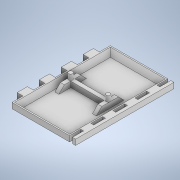
# Autodesk Inventor part: rfid_top
Saved by Autodesk Inventor 2020.1 (Build 241239000, 239)
## iProperties
Created: 2019-06-30
Part Number: rfid_top
Material: Generic
Document SubType Name: Modeling
Designer: jjsch
Density: 1 g/cm^3
Appearance: Default
Mass: 12.4406 g
Surface Area: 151.295 cm^2
Volume: 12.4406 cm^3
Author: jjsch
Autodesk Inventor part; units mm, degrees
ref_plane "YZ Plane" through (0, 0, 0) normal (1, 0, 0) x (0, 1, 0)
ref_plane "XZ Plane" through (0, 0, 0) normal (0, 1, 0) x (-1, 0, 0)
ref_plane "XY Plane" through (0, 0, 0) normal (0, 0, 1) x (1, 0, 0)
sketch "Sketch1" plane through (0, 0, 0) normal (0, 1, 0) x (-1, 0, 0)
  line L0 (-31.9185, 45) -> (31.9185, 45)
  line L1 (31.9185, 45) -> (31.9185, -45)
  line L2 (31.9185, -45) -> (-31.9185, -45)
  line L3 (-31.9185, -45) -> (-31.9185, 45)
  line L4 (-31.9185, 45) -> (31.9185, -45) construction
  line L5 (31.9185, 45) -> (-31.9185, -45) construction
  point P0 (0, 0)
  dimension "d0" = 63.837
  dimension "d1" = 90
  constraints: 12 end point, 2 midpoint, 2 parallel, 1 horizontal, 1 perpendicular
  measures "d0" distance of L1.end L2.end
  measures "d1" distance of L0.end L1.end
extrude "Extrusion1" add sketch "Sketch1" along normal blind 5
sketch "Sketch2" plane through (0, 5, 0) normal (0, 1, 0) x (1, 0, 0)
  line L0 (31.9185, -45) -> (31.9185, 45) projected
  line L1 (31.9185, -45) -> (26.4995, -45)
  line L2 (26.4995, -45) -> (26.4995, -35)
  line L3 (26.4995, -35) -> (31.9185, -35)
  line L4 (31.9185, -35) -> (31.9185, -45)
  line L5 (-31.9185, 45) -> (-31.9185, -45) projected
  line L6 (-31.9185, -45) -> (-26.4995, -45)
  line L7 (-26.4995, -45) -> (-26.4995, -35)
  line L8 (-26.4995, -35) -> (-31.9185, -35)
  line L9 (-31.9185, -35) -> (-31.9185, -45)
  line L10 (31.9185, -25) -> (26.4995, -25)
  line L11 (26.4995, -25) -> (26.4995, -15)
  line L12 (26.4995, -15) -> (31.9185, -15)
  line L13 (31.9185, -15) -> (31.9185, -25)
  line L14 (-31.9185, -25) -> (-26.4995, -25)
  line L15 (-26.4995, -25) -> (-26.4995, -15)
  line L16 (-26.4995, -15) -> (-31.9185, -15)
  line L17 (-31.9185, -15) -> (-31.9185, -25)
  line L18 (31.9185, -5) -> (26.4995, -5)
  line L19 (26.4995, -5) -> (26.4995, 5)
  line L20 (26.4995, 5) -> (31.9185, 5)
  line L21 (31.9185, 5) -> (31.9185, -5)
  line L22 (-31.9185, -5) -> (-26.4995, -5)
  line L23 (-26.4995, -5) -> (-26.4995, 5)
  line L24 (-26.4995, 5) -> (-31.9185, 5)
  line L25 (-31.9185, 5) -> (-31.9185, -5)
  line L26 (31.9185, 15) -> (26.4995, 15)
  line L27 (26.4995, 15) -> (26.4995, 25)
  line L28 (26.4995, 25) -> (31.9185, 25)
  line L29 (31.9185, 25) -> (31.9185, 15)
  line L30 (-31.9185, 15) -> (-26.4995, 15)
  line L31 (-26.4995, 15) -> (-26.4995, 25)
  line L32 (-26.4995, 25) -> (-31.9185, 25)
  line L33 (-31.9185, 25) -> (-31.9185, 15)
  line L34 (31.9185, 35) -> (26.4995, 35)
  line L35 (26.4995, 35) -> (26.4995, 45)
  line L36 (26.4995, 45) -> (31.9185, 45)
  line L37 (31.9185, 45) -> (31.9185, 35)
  line L38 (-31.9185, 35) -> (-26.4995, 35)
  line L39 (-26.4995, 35) -> (-26.4995, 45)
  line L40 (-26.4995, 45) -> (-31.9185, 45)
  line L41 (-31.9185, 45) -> (-31.9185, 35)
  point P0 (0, 0)
  dimension "d4" = 5.419
  dimension "d5" = 10
  dimension "d6" = 5.419
  dimension "d7" = 10
  dimension "d10" = 20
  constraints: 80 end point, 4 parallel, 2 horizontal, 2 perpendicular, 1 vertical, 64 other
  measures "d4" distance of L2.end L3.end
  measures "d5" distance of L1.end L2.end
  measures "d6" distance of L8.end L7.end
  measures "d7" distance of L7.end L6.end
  measures "d10" distance of L2.end L11.end
extrude "Extrusion2" cut sketch "Sketch2" against normal blind 5
sketch "Sketch3" plane through (0, 5, 0) normal (0, 1, 0) x (1, 0, 0)
  line L0 (28.4995, -45) -> (31.9185, -45)
  line L1 (31.9185, -45) -> (31.9185, 45)
  line L2 (31.9185, 45) -> (28.4995, 45)
  line L3 (28.4995, 45) -> (28.4995, -45)
  line L4 (-26.4995, -45) -> (26.4995, -45) projected
  line L5 (26.4995, -45) -> (26.4995, -35) projected
  point P0 (0, 0)
  dimension "d17" = 90
  dimension "d18" = 3.419
  dimension "d19" = 0
  dimension "d20" = 2
  constraints: 8 end point, 2 parallel, 1 horizontal, 1 perpendicular
  measures "d17" distance of L1.end L0.end
  measures "d18" distance of L0.start L0.end
  measures "d19" distance between parallel lines of L4 L0
  measures "d20" distance between parallel lines of L5 L3
extrude "Extrusion3" add sketch "Sketch3" against normal blind 5
sketch "Sketch4" plane through (0, 5, 0) normal (0, 1, 0) x (1, 0, 0)
  line L0 (31.9185, -45) -> (31.9185, 45) projected
  line L1 (31.9185, 45) -> (28.4995, 45) projected
  line L2 (28.4995, 45) -> (28.4995, 35) projected
  line L3 (28.4995, 35) -> (26.4995, 35) projected
  line L4 (26.4995, 35) -> (26.4995, 45) projected
  line L5 (26.4995, 45) -> (-26.4995, 45) projected
  line L6 (-26.4995, 45) -> (-26.4995, 35) projected
  line L7 (-26.4995, 35) -> (-31.9185, 35) projected
  line L8 (-31.9185, 35) -> (-31.9185, 25) projected
  line L9 (-31.9185, 25) -> (-26.4995, 25) projected
  line L10 (-26.4995, 25) -> (-26.4995, 15) projected
  line L11 (-26.4995, 15) -> (-31.9185, 15) projected
  line L12 (-31.9185, 15) -> (-31.9185, 5) projected
  line L13 (-31.9185, 5) -> (-26.4995, 5) projected
  line L14 (-26.4995, 5) -> (-26.4995, -5) projected
  line L15 (-26.4995, -5) -> (-31.9185, -5) projected
  line L16 (-31.9185, -5) -> (-31.9185, -15) projected
  line L17 (-31.9185, -15) -> (-26.4995, -15) projected
  line L18 (-26.4995, -15) -> (-26.4995, -25) projected
  line L19 (-26.4995, -25) -> (-31.9185, -25) projected
  line L20 (-31.9185, -25) -> (-31.9185, -35) projected
  line L21 (-31.9185, -35) -> (-26.4995, -35) projected
  line L22 (-26.4995, -35) -> (-26.4995, -45) projected
  line L23 (-26.4995, -45) -> (26.4995, -45) projected
  line L24 (26.4995, -45) -> (26.4995, -35) projected
  line L25 (26.4995, -35) -> (28.4995, -35) projected
  line L26 (28.4995, -35) -> (28.4995, -45) projected
  line L27 (28.4995, -45) -> (31.9185, -45) projected
  line L28 (28.4995, 25) -> (28.4995, 15) projected
  line L29 (28.4995, 15) -> (26.4995, 15) projected
  line L30 (26.4995, 15) -> (26.4995, 25) projected
  line L31 (26.4995, 25) -> (28.4995, 25) projected
  line L32 (28.4995, 5) -> (28.4995, -5) projected
  line L33 (28.4995, -5) -> (26.4995, -5) projected
  line L34 (26.4995, -5) -> (26.4995, 5) projected
  line L35 (26.4995, 5) -> (28.4995, 5) projected
  line L36 (28.4995, -15) -> (28.4995, -25) projected
  line L37 (28.4995, -25) -> (26.4995, -25) projected
  line L38 (26.4995, -25) -> (26.4995, -15) projected
  line L39 (26.4995, -15) -> (28.4995, -15) projected
  line L40 (-20.9995, 39.5) -> (20.9995, 39.5)
  line L41 (20.9995, 39.5) -> (20.9995, 29.5)
  line L42 (20.9995, 29.5) -> (26.4185, 29.5)
  line L43 (26.4185, 29.5) -> (26.4185, -29.5)
  line L44 (26.4185, -29.5) -> (20.9995, -29.5)
  line L45 (20.9995, -29.5) -> (20.9995, -39.5)
  line L46 (20.9995, -39.5) -> (-20.9995, -39.5)
  line L47 (-20.9995, -39.5) -> (-20.9995, -30.5)
  line L48 (-20.9995, -30.5) -> (-20.9995, -10.5)
  line L49 (-20.9995, -10.5) -> (-20.9995, 9.5)
  line L50 (-20.9995, 9.5) -> (-20.9995, 29.5)
  line L51 (-20.9995, 29.5) -> (-20.9995, 39.5)
  line L52 (20.9995, 29.5) -> (20.9995, -29.5)
  point P0 (0, 0)
  dimension "d23" = 5.5
  constraints: 26 end point, 1 collinear, 11 other
  measures "d23" distance between parallel lines of L5 L40
extrude "Extrusion4" cut sketch "Sketch4" against normal blind 4 contours L40 L41 L52 L45 L46 L47 L48 L49 L50 L51
chamfer "Chamfer1" distance 4 angle 45 4 edges at (-20.9995, 5, 0) (0, 5, -39.5) (20.9995, 5, 0) (0, 5, 39.5)
sketch "Sketch9" plane through (0, 5, 0) normal (0, 1, 0) x (1, 0, 0)
  line L0 (28.4995, -15) -> (28.4995, -25) projected
  line L1 (28.4995, -25) -> (26.4995, -25) projected
  line L2 (26.4995, -25) -> (26.4995, -15) projected
  line L3 (26.4995, -15) -> (28.4995, -15) projected
  line L4 (28.4995, 5) -> (28.4995, -5) projected
  line L5 (28.4995, -5) -> (26.4995, -5) projected
  line L6 (26.4995, -5) -> (26.4995, 5) projected
  line L7 (26.4995, 5) -> (28.4995, 5) projected
  line L8 (28.4995, 25) -> (28.4995, 15) projected
  line L9 (28.4995, 15) -> (26.4995, 15) projected
  line L10 (26.4995, 15) -> (26.4995, 25) projected
  line L11 (26.4995, 25) -> (28.4995, 25) projected
  line L12 (31.9185, -45) -> (31.9185, 45) projected
  line L13 (31.9185, 45) -> (28.4995, 45) projected
  line L14 (28.4995, 45) -> (28.4995, 35) projected
  line L15 (28.4995, 35) -> (26.4995, 35) projected
  line L16 (26.4995, 35) -> (26.4995, 45) projected
  line L17 (26.4995, 45) -> (-26.4995, 45) projected
  line L18 (-26.4995, 45) -> (-26.4995, 35) projected
  line L19 (-26.4995, 35) -> (-31.9185, 35) projected
  line L20 (-31.9185, 35) -> (-31.9185, 25) projected
  line L21 (-31.9185, 25) -> (-26.4995, 25) projected
  line L22 (-26.4995, 25) -> (-26.4995, 15) projected
  line L23 (-26.4995, 15) -> (-31.9185, 15) projected
  line L24 (-31.9185, 15) -> (-31.9185, 5) projected
  line L25 (-31.9185, 5) -> (-26.4995, 5) projected
  line L26 (-26.4995, 5) -> (-26.4995, -5) projected
  line L27 (-26.4995, -5) -> (-31.9185, -5) projected
  line L28 (-31.9185, -5) -> (-31.9185, -15) projected
  line L29 (-31.9185, -15) -> (-26.4995, -15) projected
  line L30 (-26.4995, -15) -> (-26.4995, -25) projected
  line L31 (-26.4995, -25) -> (-31.9185, -25) projected
  line L32 (-31.9185, -25) -> (-31.9185, -35) projected
  line L33 (-31.9185, -35) -> (-26.4995, -35) projected
  line L34 (-26.4995, -35) -> (-26.4995, -45) projected
  line L35 (-26.4995, -45) -> (26.4995, -45) projected
  line L36 (26.4995, -45) -> (26.4995, -35) projected
  line L37 (26.4995, -35) -> (28.4995, -35) projected
  line L38 (28.4995, -35) -> (28.4995, -45) projected
  line L39 (28.4995, -45) -> (31.9185, -45) projected
  line L40 (24.9995, 43.5) -> (-24.9995, 43.5) projected
  line L41 (24.9995, -43.5) -> (24.9995, 43.5) projected
  line L42 (-24.9995, -43.5) -> (24.9995, -43.5) projected
  line L43 (-24.9995, 43.5) -> (-24.9995, -43.5) projected
  line L44 (31.6185, 44.7) -> (31.6185, -44.7)
  line L45 (31.6185, -44.7) -> (28.7995, -44.7)
  line L46 (28.7995, -44.7) -> (28.7995, -34.7)
  line L47 (28.7995, -34.7) -> (26.1995, -34.7)
  line L48 (26.1995, -34.7) -> (26.1995, -44.7)
  line L49 (26.1995, -44.7) -> (-26.1995, -44.7)
  line L50 (-26.1995, -44.7) -> (-26.1995, -34.7)
  line L51 (-26.1995, -34.7) -> (-31.6185, -34.7)
  line L52 (-31.6185, -34.7) -> (-31.6185, -25.3)
  line L53 (-31.6185, -25.3) -> (-26.1995, -25.3)
  line L54 (-26.1995, -25.3) -> (-26.1995, -14.7)
  line L55 (-26.1995, -14.7) -> (-31.6185, -14.7)
  line L56 (-31.6185, -14.7) -> (-31.6185, -5.3)
  line L57 (-31.6185, -5.3) -> (-26.1995, -5.3)
  line L58 (-26.1995, -5.3) -> (-26.1995, 5.3)
  line L59 (-26.1995, 5.3) -> (-31.6185, 5.3)
  line L60 (-31.6185, 5.3) -> (-31.6185, 14.7)
  line L61 (-31.6185, 14.7) -> (-26.1995, 14.7)
  line L62 (-26.1995, 14.7) -> (-26.1995, 25.3)
  line L63 (-26.1995, 25.3) -> (-31.6185, 25.3)
  line L64 (-31.6185, 25.3) -> (-31.6185, 34.7)
  line L65 (-31.6185, 34.7) -> (-26.1995, 34.7)
  line L66 (-26.1995, 34.7) -> (-26.1995, 44.7)
  line L67 (-26.1995, 44.7) -> (26.1995, 44.7)
  line L68 (26.1995, 44.7) -> (26.1995, 34.7)
  line L69 (26.1995, 34.7) -> (28.7995, 34.7)
  line L70 (28.7995, 34.7) -> (28.7995, 44.7)
  line L71 (28.7995, 44.7) -> (31.6185, 44.7)
  line L72 (28.7995, -25.3) -> (28.7995, -14.7)
  line L73 (28.7995, -14.7) -> (26.1995, -14.7)
  line L74 (26.1995, -14.7) -> (26.1995, -25.3)
  line L75 (26.1995, -25.3) -> (28.7995, -25.3)
  line L76 (28.7995, -5.3) -> (28.7995, 5.3)
  line L77 (28.7995, 5.3) -> (26.1995, 5.3)
  line L78 (26.1995, 5.3) -> (26.1995, -5.3)
  line L79 (26.1995, -5.3) -> (28.7995, -5.3)
  line L80 (26.1995, 25.3) -> (26.1995, 14.7)
  line L81 (26.1995, 14.7) -> (28.7995, 14.7)
  line L82 (28.7995, 14.7) -> (28.7995, 25.3)
  line L83 (28.7995, 25.3) -> (26.1995, 25.3)
  line L84 (28.4995, -15) -> (28.4995, -25) projected
  line L85 (28.4995, -25) -> (26.4995, -25) projected
  line L86 (26.4995, -25) -> (26.4995, -15) projected
  line L87 (26.4995, -15) -> (28.4995, -15) projected
  line L88 (28.4995, 5) -> (28.4995, -5) projected
  line L89 (28.4995, -5) -> (26.4995, -5) projected
  line L90 (26.4995, -5) -> (26.4995, 5) projected
  line L91 (26.4995, 5) -> (28.4995, 5) projected
  line L92 (28.4995, 25) -> (28.4995, 15) projected
  line L93 (28.4995, 15) -> (26.4995, 15) projected
  line L94 (26.4995, 15) -> (26.4995, 25) projected
  line L95 (26.4995, 25) -> (28.4995, 25) projected
  line L96 (31.9185, -45) -> (31.9185, 45) projected
  line L97 (31.9185, 45) -> (28.4995, 45) projected
  line L98 (28.4995, 45) -> (28.4995, 35) projected
  line L99 (28.4995, 35) -> (26.4995, 35) projected
  line L100 (26.4995, 35) -> (26.4995, 45) projected
  line L101 (26.4995, 45) -> (-26.4995, 45) projected
  line L102 (-26.4995, 45) -> (-26.4995, 35) projected
  line L103 (-26.4995, 35) -> (-31.9185, 35) projected
  line L104 (-31.9185, 35) -> (-31.9185, 25) projected
  line L105 (-31.9185, 25) -> (-26.4995, 25) projected
  line L106 (-26.4995, 25) -> (-26.4995, 15) projected
  line L107 (-26.4995, 15) -> (-31.9185, 15) projected
  line L108 (-31.9185, 15) -> (-31.9185, 5) projected
  line L109 (-31.9185, 5) -> (-26.4995, 5) projected
  line L110 (-26.4995, 5) -> (-26.4995, -5) projected
  line L111 (-26.4995, -5) -> (-31.9185, -5) projected
  line L112 (-31.9185, -5) -> (-31.9185, -15) projected
  line L113 (-31.9185, -15) -> (-26.4995, -15) projected
  line L114 (-26.4995, -15) -> (-26.4995, -25) projected
  line L115 (-26.4995, -25) -> (-31.9185, -25) projected
  line L116 (-31.9185, -25) -> (-31.9185, -35) projected
  line L117 (-31.9185, -35) -> (-26.4995, -35) projected
  line L118 (-26.4995, -35) -> (-26.4995, -45) projected
  line L119 (-26.4995, -45) -> (26.4995, -45) projected
  line L120 (26.4995, -45) -> (26.4995, -35) projected
  line L121 (26.4995, -35) -> (28.4995, -35) projected
  line L122 (28.4995, -35) -> (28.4995, -45) projected
  line L123 (28.4995, -45) -> (31.9185, -45) projected
  line L124 (24.9995, 43.5) -> (-24.9995, 43.5) projected
  line L125 (24.9995, -43.5) -> (24.9995, 43.5) projected
  line L126 (-24.9995, -43.5) -> (24.9995, -43.5) projected
  line L127 (-24.9995, 43.5) -> (-24.9995, -43.5) projected
  point P0 (0, 0)
  dimension "d55" = 0.3
  dimension "d56" = 0.3
  dimension "d57" = 0.3
  dimension "d58" = 0.3
  constraints: 80 end point, 36 other
  measures "d55" distance between parallel lines of L12 L44
  measures "d56" distance between parallel lines of L0 L72
  measures "d57" distance between parallel lines of L4 L76
  measures "d58" distance between parallel lines of L10 L80
extrude "Tolerances Extrusion" cut sketch "Sketch9" against normal blind 5 contours L0 L1 L2 L3 | L4 L5 L6 L7 | L8 L9 L10 L11 | L39 L38 L37 L36 L35 L34 L33 L32 L31 L30 L29 L28 L27 L26 L25 L24 L23 L22 L21 L20 L19 L18 L17 L16 L15 L14 L13 L12 | L75 L74 L73 L72 | L79 L78 L77 L76 | L83 L82 L81 L80
sketch "Sketch11" plane through (0, 1, 0) normal (0, 1, 0) x (1, 0, 0)
  line L0 (0, 0) -> (0, 21.734)
  circle A0 centre (-17.05, -0.5) radius 1.825
  circle A1 centre (17.05, -0.5) radius 1.825
  line L1 (-26.1995, -44.7) -> (26.1995, -44.7) projected
  dimension "d76" = 3.65
  dimension "d77" = 3.65
  dimension "d78" = 17.05
  dimension "d79" = 17.05
  dimension "d80" = 44.2
  dimension "d81" = 44.2
  constraints: 2 centre point, 2 end point, 1 vertical
  measures "d76" diameter of A0
  measures "d77" diameter of A1
  measures "d78" distance from line of L0 A0.centre
  measures "d79" distance from line of A1.centre L0
  measures "d80" distance from line of L1 A1.centre
  measures "d81" distance from line of L1 A0.centre
extrude "Extrusion10" add sketch "Sketch11" along normal blind 10
sketch "Sketch12" plane through (0, 1, 0) normal (0, 1, 0) x (1, 0, 0)
  circle A0 centre (17.05, -0.5) radius 1.825 projected
  circle A1 centre (-17.05, -0.5) radius 1.825 projected
  circle A2 centre (17.05, -0.5) radius 1.825 projected
  line L0 (17.05, -0.5) -> (-17.05, -0.5)
  line L1 (-17.05, -2.325) -> (17.05, -2.325)
  line L2 (17.05, -2.325) -> (17.05, 1.325)
  line L3 (17.05, 1.325) -> (-17.05, 1.325)
  line L4 (-17.05, 1.325) -> (-17.05, -2.325)
  line L5 (-17.05, -2.325) -> (17.05, 1.325) construction
  line L6 (17.05, -2.325) -> (-17.05, 1.325) construction
  line L7 (-18.875, -13) -> (-15.225, -13)
  line L8 (-15.225, -13) -> (-15.225, 12)
  line L9 (-15.225, 12) -> (-18.875, 12)
  line L10 (-18.875, 12) -> (-18.875, -13)
  line L11 (-18.875, -13) -> (-15.225, 12) construction
  line L12 (-15.225, -13) -> (-18.875, 12) construction
  line L13 (15.225, -13) -> (18.875, -13)
  line L14 (18.875, -13) -> (18.875, 12)
  line L15 (18.875, 12) -> (15.225, 12)
  line L16 (15.225, 12) -> (15.225, -13)
  line L17 (15.225, -13) -> (18.875, 12) construction
  line L18 (18.875, -13) -> (15.225, 12) construction
  point P0 (0, 0)
  point P1 (17.3644, 0.2709)
  point P2 (0, -0.5)
  point P3 (-18.875, -0.5)
  point P4 (-15.225, -2.325)
  point P5 (15.225, -2.325)
  point P6 (18.875, -0.5)
  point P7 (15.225, 1.325)
  point P8 (-15.225, 1.325)
  dimension "d84" = 25
  dimension "d85" = 25
  constraints: 38 end point, 7 midpoint, 6 parallel, 4 horizontal, 3 perpendicular, 2 coincident, 1 vertical alignment, 1 other
  measures "d84" distance of L8.end L7.end
  measures "d85" distance of L14.end L13.end
extrude "Extrusion11" add sketch "Sketch12" along normal blind 5 contours L14 L13 L16 L1 A0 | A0 L3 L16 L15 L14 | L2 L0 A0 | A0 L16 L3 | L1 L16 A0 | A0 L0 L2 | L16 L1 L8 L0 | L0 L8 L3 L16 | L0 L4 A1 | L8 L1 A1 | A1 L4 L0 | A1 L3 L8 | L3 A1 L10 L9 L8 | L8 L7 L10 A1 L1
chamfer "Chamfer3" distance 5 angle 45 4 edges at (17.05, 6, -12) (17.05, 6, 13) (-17.05, 6, -12) (-17.05, 6, 13)
sketch "Sketch13" plane through (0, 0, 0) normal (0, -1, 0) x (1, 0, 0)
  line L0 (26.1995, -5.3) -> (26.1995, 5.3) projected
  line L1 (26.1995, 5.3) -> (28.7995, 5.3) projected
  line L2 (28.7995, 5.3) -> (28.7995, -5.3) projected
  line L3 (28.7995, -5.3) -> (26.1995, -5.3) projected
  line L4 (28.7995, 14.7) -> (26.1995, 14.7) projected
  line L5 (26.1995, 14.7) -> (26.1995, 25.3) projected
  line L6 (26.1995, 25.3) -> (28.7995, 25.3) projected
  line L7 (28.7995, 25.3) -> (28.7995, 14.7) projected
  line L8 (26.1995, -14.7) -> (28.7995, -14.7) projected
  line L9 (28.7995, -14.7) -> (28.7995, -25.3) projected
  line L10 (28.7995, -25.3) -> (26.1995, -25.3) projected
  line L11 (26.1995, -25.3) -> (26.1995, -14.7) projected
  line L12 (26.1995, 34.7) -> (26.1995, 44.7) projected
  line L13 (26.1995, 44.7) -> (-26.1995, 44.7) projected
  line L14 (-26.1995, 44.7) -> (-26.1995, 34.7) projected
  line L15 (-26.1995, 34.7) -> (-31.6185, 34.7) projected
  line L16 (-31.6185, 34.7) -> (-31.6185, 25.3) projected
  line L17 (-31.6185, 25.3) -> (-26.1995, 25.3) projected
  line L18 (-26.1995, 25.3) -> (-26.1995, 14.7) projected
  line L19 (-26.1995, 14.7) -> (-31.6185, 14.7) projected
  line L20 (-31.6185, 14.7) -> (-31.6185, 5.3) projected
  line L21 (-31.6185, 5.3) -> (-26.1995, 5.3) projected
  line L22 (-26.1995, 5.3) -> (-26.1995, -5.3) projected
  line L23 (-26.1995, -5.3) -> (-31.6185, -5.3) projected
  line L24 (-31.6185, -5.3) -> (-31.6185, -14.7) projected
  line L25 (-31.6185, -14.7) -> (-26.1995, -14.7) projected
  line L26 (-26.1995, -14.7) -> (-26.1995, -25.3) projected
  line L27 (-26.1995, -25.3) -> (-31.6185, -25.3) projected
  line L28 (-31.6185, -25.3) -> (-31.6185, -34.7) projected
  line L29 (-31.6185, -34.7) -> (-26.1995, -34.7) projected
  line L30 (-26.1995, -34.7) -> (-26.1995, -44.7) projected
  line L31 (-26.1995, -44.7) -> (26.1995, -44.7) projected
  line L32 (26.1995, -44.7) -> (26.1995, -34.7) projected
  line L33 (26.1995, -34.7) -> (28.7995, -34.7) projected
  line L34 (28.7995, -34.7) -> (28.7995, -44.7) projected
  line L35 (28.7995, -44.7) -> (31.6185, -44.7) projected
  line L36 (31.6185, -44.7) -> (31.6185, 44.7) projected
  line L37 (31.6185, 44.7) -> (28.7995, 44.7) projected
  line L38 (28.7995, 44.7) -> (28.7995, 34.7) projected
  line L39 (28.7995, 34.7) -> (26.1995, 34.7) projected
  line L40 (26.1995, -44.7) -> (-26.1995, -44.7) projected
  line L41 (-26.1995, -44.7) -> (26.1995, -44.7)
  line L42 (26.1995, -44.7) -> (26.1995, -46.7)
  line L43 (26.1995, -46.7) -> (-26.1995, -46.7)
  line L44 (-26.1995, -46.7) -> (-26.1995, -44.7)
  line L45 (-26.1995, 44.7) -> (-26.1995, 34.7) projected
  line L46 (-26.1995, 44.7) -> (26.1995, 44.7)
  line L47 (26.1995, 44.7) -> (26.1995, 46.7)
  line L48 (26.1995, 46.7) -> (-26.1995, 46.7)
  line L49 (-26.1995, 46.7) -> (-26.1995, 44.7)
  point P0 (0, 0)
  point P1 (26.1995, -45.7)
  dimension "d91" = 2
  dimension "d92" = 2
  constraints: 16 end point, 4 parallel, 2 horizontal, 2 perpendicular, 1 midpoint, 1 point on line
  measures "d91" distance of L41.end L42.end
  measures "d92" distance of L47.end L46.end
extrude "Extrusion12" add sketch "Sketch13" against normal up to surface (5 mm away) contours L13 L49 L48 L47 | L42 L43 L44 L31
sketch "Sketch14" plane through (0, 0, 0) normal (0, -1, 0) x (1, 0, 0)
  line L0 (26.1995, -5.3) -> (26.1995, 5.3) projected
  line L1 (26.1995, 5.3) -> (28.7995, 5.3) projected
  line L2 (28.7995, 5.3) -> (28.7995, -5.3) projected
  line L3 (28.7995, -5.3) -> (26.1995, -5.3) projected
  line L4 (28.7995, 14.7) -> (26.1995, 14.7) projected
  line L5 (26.1995, 14.7) -> (26.1995, 25.3) projected
  line L6 (26.1995, 25.3) -> (28.7995, 25.3) projected
  line L7 (28.7995, 25.3) -> (28.7995, 14.7) projected
  line L8 (26.1995, -14.7) -> (28.7995, -14.7) projected
  line L9 (28.7995, -14.7) -> (28.7995, -25.3) projected
  line L10 (28.7995, -25.3) -> (26.1995, -25.3) projected
  line L11 (26.1995, -25.3) -> (26.1995, -14.7) projected
  line L12 (26.1995, 34.7) -> (26.1995, 46.7) projected
  line L13 (26.1995, 46.7) -> (-26.1995, 46.7) projected
  line L14 (-26.1995, 46.7) -> (-26.1995, 34.7) projected
  line L15 (-26.1995, 34.7) -> (-31.6185, 34.7) projected
  line L16 (-31.6185, 34.7) -> (-31.6185, 25.3) projected
  line L17 (-31.6185, 25.3) -> (-26.1995, 25.3) projected
  line L18 (-26.1995, 25.3) -> (-26.1995, 14.7) projected
  line L19 (-26.1995, 14.7) -> (-31.6185, 14.7) projected
  line L20 (-31.6185, 14.7) -> (-31.6185, 5.3) projected
  line L21 (-31.6185, 5.3) -> (-26.1995, 5.3) projected
  line L22 (-26.1995, 5.3) -> (-26.1995, -5.3) projected
  line L23 (-26.1995, -5.3) -> (-31.6185, -5.3) projected
  line L24 (-31.6185, -5.3) -> (-31.6185, -14.7) projected
  line L25 (-31.6185, -14.7) -> (-26.1995, -14.7) projected
  line L26 (-26.1995, -14.7) -> (-26.1995, -25.3) projected
  line L27 (-26.1995, -25.3) -> (-31.6185, -25.3) projected
  line L28 (-31.6185, -25.3) -> (-31.6185, -34.7) projected
  line L29 (-31.6185, -34.7) -> (-26.1995, -34.7) projected
  line L30 (-26.1995, -34.7) -> (-26.1995, -46.7) projected
  line L31 (-26.1995, -46.7) -> (26.1995, -46.7) projected
  line L32 (26.1995, -46.7) -> (26.1995, -34.7) projected
  line L33 (26.1995, -34.7) -> (28.7995, -34.7) projected
  line L34 (28.7995, -34.7) -> (28.7995, -44.7) projected
  line L35 (28.7995, -44.7) -> (31.6185, -44.7) projected
  line L36 (31.6185, -44.7) -> (31.6185, 44.7) projected
  line L37 (31.6185, 44.7) -> (28.7995, 44.7) projected
  line L38 (28.7995, 44.7) -> (28.7995, 34.7) projected
  line L39 (28.7995, 34.7) -> (26.1995, 34.7) projected
  line L40 (26.1995, 34.7) -> (26.1995, 46.7) projected
  line L41 (-26.1995, 46.7) -> (-26.1995, 34.7) projected
  line L42 (26.1995, 44.7) -> (-26.1995, 44.7)
  line L43 (-26.1995, 46.7) -> (-26.1995, 34.7) projected
  line L44 (0, 0) -> (13.9667, 0)
  line L45 (26.1995, 46.7) -> (-26.1995, 46.7) projected
  line L46 (26.1995, 44.7) -> (-26.1995, 44.7)
  line L47 (-26.1995, 44.7) -> (-26.1995, 46.7)
  line L48 (-26.1995, 46.7) -> (26.1995, 46.7)
  line L49 (26.1995, 46.7) -> (26.1995, 44.7)
  line L50 (26.1995, -46.7) -> (26.1995, -34.7) projected
  line L51 (-26.1995, -46.7) -> (-26.1995, -34.7) projected
  line L52 (26.1995, -44.7) -> (-26.1995, -44.7)
  line L53 (-26.1995, -44.7) -> (-26.1995, -46.7)
  line L54 (-26.1995, -46.7) -> (26.1995, -46.7)
  line L55 (26.1995, -46.7) -> (26.1995, -44.7)
  point P0 (-26.1995, -44.7)
  constraints: 20 end point, 4 parallel, 3 horizontal, 3 perpendicular, 3 point on line
extrude "Extrusion13" cut sketch "Sketch14" against normal blind 10 contours L42 L14 L13 L12 | L32 L31 L30 L52
body "Solid1"
